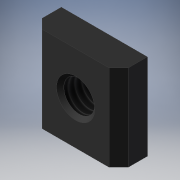
# Autodesk Inventor part: 14159_m
Saved by Autodesk Inventor 2019 (Build 230136000, 136)
## iProperties
Created: 2024-04-27
Part Number: 14159_m
Material: Generic
Catalog Web Link: www.cadenas.de
Description: 14159, 14122, 14124, 14126, 14127, 14128, 14129, 14130, 14131_m-Slide-In Economy T-Nuts
Vendor: 8020
Document SubType Name: Modeling
Designer: psAdmin
Manufacturer: 8020
Mass: 0.207658 g
Surface Area: 2.67352 cm^2
Volume: 0.207658 cm^3
Density: 1 g/cm^3
Appearance: PSOLRGB-175-175-175
Category: PARTsolutions
Company: 8020
Title: 14159
Author: Cadenas PARTsolutions
Comments: Slide-In Economy T-Nuts
PSOL_IDENT_0: {$CADENAS_DATA/23d-libs/8020/metric/fastening_options/14159_m.prj},209 {VTYP=3D},{NB=14159_m},{LINA=
PSOL_IDENT_1: 14159},{NN=14159, 14122, 14124, 14126, 14127, 14128, 14129, 14130, 14131_m},{DATE=09.11.2023 07:10:0
PSOL_IDENT_2: 6},{GEOMDATE=20.06.2019 14:19:00},{VERSION=},{LINEID=10},{WBVAR=},{WBNUMERIC=}  {NB=14159_m},{LINA=1
PSOL_IDENT_3: 4159},{KT=DUMMY},{PN=14159},{MAT=Steel},{FIN=Zinc-Plated},{A=M4},{A1=4},{B=9.00},{C=9.00},{D=3.00},{
PSOL_IDENT_4: CC=5-20}
NB: 14159_m
NN: 14159, 14122, 14124, 14126, 14127, 14128, 14129, 14130, 14131_m
NT: Slide-In Economy T-Nuts
NBSYN: $PN._m
LINA: 14159
CATALOG: 80/20
PN: 14159
MAT: Steel
FIN: Zinc-Plated
A: M4
B: 9
C: 9
D: 3
CC: 5-20
SUPPLIER: 8020
ARTICLENO: 14159_m
BOMINFO: 14159
CREATOR: CADENAS GmbH
Autodesk Inventor part; units mm, degrees
ref_plane "YZ Plane" through (0, 0, 0) normal (1, 0, 0) x (0, 1, 0)
ref_plane "XZ Plane" through (0, 0, 0) normal (0, 1, 0) x (-1, 0, 0)
ref_plane "XY Plane" through (0, 0, 0) normal (0, 0, 1) x (1, 0, 0)
sketch "Sketch_1" plane through (0, 0, 0) normal (0, 0, 1) x (1, 0, 0)
  line L0 (-4.5, 4.5) -> (-4.5, -4.5)
  line L1 (-4.5, -4.5) -> (4.5, -4.5)
  line L2 (4.5, -4.5) -> (4.5, 4.5)
  line L3 (4.5, 4.5) -> (-4.5, 4.5)
  constraints: 8 end point
extrude "Extrusion1" add sketch "Sketch_1" along normal mid plane 3
sketch "Sketch_2" plane through (0, 0, 0) normal (1, 0, 0) x (0, 1, 0)
  line L0 (0, -1.5) -> (0, 1.5)
  line L1 (0, 1.5) -> (2, 1.5)
  line L2 (2, 1.5) -> (1.621, 1.121)
  line L3 (1.621, 1.121) -> (1.621, -1.121)
  line L4 (1.621, -1.121) -> (2, -1.5)
  line L5 (2, -1.5) -> (0, -1.5)
  line L6 (0, -1.5) -> (0, 1.5)
  constraints: 14 end point
revolve "Revolution1" cut sketch "Sketch_2" angle 360 about axis through (0, 0, -1.5) along (0, 0, -1)
thread "Thread1" size "M4x0.7" class "6H" standard "ISO Metric profile" full length
sketch "Sketch_3" plane through (0, 0, 0) normal (0, 1, 0) x (-1, 0, 0)
  line L0 (4.5, 0.5) -> (4.5, 2.5)
  line L1 (4.5, 2.5) -> (-4.5, 2.5)
  line L2 (-4.5, 2.5) -> (-4.5, 0.5)
  line L3 (-4.5, 0.5) -> (-3.5, 1.5)
  line L4 (-3.5, 1.5) -> (3.5, 1.5)
  line L5 (3.5, 1.5) -> (4.5, 0.5)
  constraints: 12 end point
extrude "Extrusion2" cut sketch "Sketch_3" along normal mid plane 18
body "Solid1"
